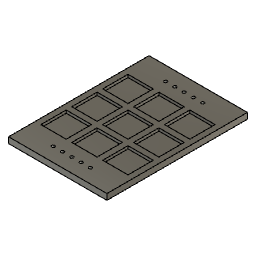
Verkefni_4 (v2~recovered) (Autodesk Fusion 360 design; units mm, degrees)
Autodesk Fusion 360 part; units mm, degrees
sketch "Sketch1" plane through (0, 0, 0) normal (0, 0, 1) x (1, 0, 0)
  line L0 (0, 0) -> (0, 500)
  line L1 (0, 500) -> (350, 500)
  line L2 (350, 500) -> (350, 0)
  line L3 (350, 0) -> (0, 0)
  dimension "d6" = 500
  dimension "d7" = 350
  dimension "d8" = 500
  dimension "d9" = 350
  constraint coincident L0.start L3.end
  constraint vertical L0
  constraint perpendicular L0 L1
  constraint perpendicular L1 L2
  measures "d6" distance of L0.start L0.end
  measures "d7" distance of L0.end L1.end
  measures "d8" distance of L1.end L2.end
  measures "d9" distance of L2.end L0.start
extrude "Extrude1" add sketch "Sketch1" along normal blind 21
sketch "Sketch2" plane through (0, 0, 21) normal (0, 0, 1) x (-1, 0, 0)
  line L0 (-350, 0) -> (-350, -500)
  line L1 (-350, -500) -> (0, -500)
  line L2 (0, -500) -> (0, 0)
  line L3 (0, 0) -> (-350, 0)
  line L4 (0, 0) -> (-20, 0)
  line L5 (-350, 0) -> (-330, 0)
  line L6 (-330, 0) -> (-330, -500)
  line L7 (-20, 0) -> (-20, -500)
  line L8 (-20, -500) -> (-110, -500)
  line L9 (-110, -500) -> (-130, -500)
  line L10 (-130, -500) -> (-220, -500)
  line L11 (-220, -500) -> (-240, -500)
  line L12 (-240, -500) -> (-330, -500)
  line L13 (-110, -500) -> (-110, 0)
  line L14 (-130, -500) -> (-130, 0)
  line L15 (-220, -500) -> (-220, 0)
  line L16 (-240, -500) -> (-240, 0)
  line L17 (0, 0) -> (0, -95)
  line L18 (0, -500) -> (0, -405)
  line L19 (0, -405) -> (-350, -405)
  line L20 (0, -95) -> (-350, -95)
  line L21 (0, -405) -> (0, -315)
  line L22 (0, -315) -> (0, -295)
  line L23 (0, -295) -> (0, -205)
  line L24 (0, -205) -> (0, -185)
  line L25 (0, -185) -> (0, -95)
  line L26 (0, -185) -> (-350, -185)
  line L27 (0, -205) -> (-350, -205)
  line L28 (0, -295) -> (-350, -295)
  line L29 (0, -315) -> (-350, -315)
  dimension "d13" = 20
  dimension "d14" = 500
  dimension "d16" = 90
  dimension "d19" = 20
  dimension "d27" = 95
  dimension "d28" = 95
  dimension "d29" = 350
  dimension "d31" = 90
  dimension "d32" = 20
  dimension "d34" = 90
  dimension "d35" = 20
  constraint coincident L2.end L3.start
  constraint coincident L3 L4.end
  constraint coincident L0.start L3.end
  constraint coincident L3 L5.end
  constraint vertical L6
  constraint vertical L7
  constraint perpendicular L7 L8
  constraint perpendicular L7 L9
  constraint perpendicular L7 L10
  constraint parallel L1 L11
  constraint parallel L1 L12
  constraint perpendicular L9 L13
  constraint perpendicular L8 L14
  constraint perpendicular L1 L15
  constraint perpendicular L11 L16
  constraint parallel L2 L17
  constraint coincident L1.end L2.start
  constraint perpendicular L1 L18
  constraint perpendicular L0 L19
  constraint perpendicular L0 L20
  constraint perpendicular L19 L21
  constraint parallel L2 L22
  constraint coincident L2 L23.end
  constraint coincident L2 L24.end
  constraint coincident L0 L26.end
  constraint perpendicular L0 L26
  constraint coincident L0 L27.end
  constraint perpendicular L0 L27
  constraint coincident L0 L28.end
  constraint perpendicular L0 L28
  constraint coincident L0 L29.end
  constraint perpendicular L0 L29
  measures "d13" distance of L0.start L5.end
  measures "d14" distance of L5.end L6.end
  measures "d16" distance of L7.end L8.end
  measures "d19" distance of L10.end L11.end
  measures "d27" distance of L2.end L17.end
  measures "d28" distance of L1.end L18.end
  measures "d29" distance of L18.end L19.end
  measures "d31" distance of L18.end L21.end
  measures "d32" distance of L21.end L22.end
  measures "d34" distance of L22.end L23.end
  measures "d35" distance of L23.end L24.end
extrude "Extrude2" cut sketch "Sketch2" against normal blind 10 contours L6 L16 L20 L26 | L6 L16 L27 L28 | L14 L15 L20 L26 | L6 L16 L19 L29 | L14 L15 L27 L28 | L7 L13 L20 L26 | L14 L15 L19 L29 | L7 L13 L27 L28 | L7 L13 L19 L29
sketch "Sketch3" plane through (0, 0, 21) normal (0, 0, 1) x (-1, 0, 0)
  line L0 (-330, -95) -> (-240, -95)
  line L1 (-240, -95) -> (-240, -185)
  line L2 (-240, -185) -> (-330, -185)
  line L3 (-330, -185) -> (-330, -95)
  line L4 (-130, -205) -> (-130, -295)
  line L5 (-130, -295) -> (-220, -295)
  line L6 (-220, -295) -> (-220, -205)
  line L7 (-220, -205) -> (-130, -205)
  line L8 (-110, -405) -> (-110, -315)
  line L9 (-110, -315) -> (-20, -315)
  line L10 (-20, -315) -> (-20, -405)
  line L11 (-20, -405) -> (-110, -405)
  line L12 (-110, -295) -> (-110, -205)
  line L13 (-110, -205) -> (-20, -205)
  line L14 (-20, -205) -> (-20, -295)
  line L15 (-20, -295) -> (-110, -295)
  line L16 (-130, -95) -> (-130, -185)
  line L17 (-130, -185) -> (-220, -185)
  line L18 (-220, -185) -> (-220, -95)
  line L19 (-220, -95) -> (-130, -95)
  line L20 (-330, -205) -> (-240, -205)
  line L21 (-240, -205) -> (-240, -295)
  line L22 (-240, -295) -> (-330, -295)
  line L23 (-330, -295) -> (-330, -205)
  line L24 (-130, -315) -> (-130, -405)
  line L25 (-130, -405) -> (-220, -405)
  line L26 (-220, -405) -> (-220, -315)
  line L27 (-220, -315) -> (-130, -315)
  line L28 (-330, -315) -> (-240, -315)
  line L29 (-240, -315) -> (-240, -405)
  line L30 (-240, -405) -> (-330, -405)
  line L31 (-330, -405) -> (-330, -315)
  line L32 (-110, -185) -> (-110, -95)
  line L33 (-110, -95) -> (-20, -95)
  line L34 (-20, -95) -> (-20, -185)
  line L35 (-20, -185) -> (-110, -185)
  line L36 (0, 0) -> (-175, 0)
  circle A0 centre (-175, -50) radius 5.5
  circle A1 centre (-208, -50) radius 5.5
  circle A2 centre (-241, -50) radius 5.5
  circle A3 centre (-142, -50) radius 5.5
  circle A4 centre (-109, -50) radius 5.5
  line L37 (0, -500) -> (-175, -500)
  circle A5 centre (-142, -450) radius 5.5
  circle A6 centre (-109, -450) radius 5.5
  circle A7 centre (-208, -450) radius 5.5
  circle A8 centre (-175, -450) radius 5.5
  circle A9 centre (-241, -450) radius 5.5
  line L38 (-350, 0) -> (-350, -500)
  line L39 (-350, -500) -> (0, -500)
  line L40 (0, -500) -> (0, 0)
  line L41 (0, 0) -> (-350, 0)
  dimension "d43" = 175
  dimension "d44" = 50
  dimension "d46" = 33
  dimension "d55" = 11
  dimension "d56" = 175
  dimension "d57" = 50
  dimension "d60" = 33
  dimension "d64" = 11
  constraint horizontal L36
  constraint coincident L36.start L40.end
  constraint horizontal L37
  measures "d43" distance of L36.start L36.end
  measures "d44" distance of L36.end A0.centre
  measures "d46" distance of A0.centre A1.centre
  measures "d55" diameter of A4
  measures "d56" distance of L37.start L37.end
  measures "d57" distance of L37.end A8.centre
  measures "d60" distance of A7.centre A9.centre
  measures "d64" diameter of A6
extrude "Extrude3" cut sketch "Sketch3" against normal blind 11 contours A0 | A1 | A2 | A3 | A4 | A5 | A6 | A7 | A8 | A9
sketch "Sketch5" plane through (0, 0, 21) normal (0, 0, 1) x (-1, 0, 0)
  circle A0 centre (-175, -50) radius 5.5
  circle A1 centre (-208, -450) radius 5.5
  circle A2 centre (-109, -450) radius 5.5
  circle A3 centre (-241, -450) radius 5.5
  circle A4 centre (-208, -50) radius 5.5
  circle A5 centre (-142, -50) radius 5.5
  circle A6 centre (-175, -450) radius 5.5
  circle A7 centre (-142, -450) radius 5.5
  circle A8 centre (-109, -50) radius 5.5
  circle A9 centre (-241, -50) radius 5.5
  line L0 (-110, -185) -> (-110, -95)
  line L1 (-110, -95) -> (-20, -95)
  line L2 (-20, -95) -> (-20, -185)
  line L3 (-20, -185) -> (-110, -185)
  line L4 (-330, -315) -> (-240, -315)
  line L5 (-240, -315) -> (-240, -405)
  line L6 (-240, -405) -> (-330, -405)
  line L7 (-330, -405) -> (-330, -315)
  line L8 (-130, -315) -> (-130, -405)
  line L9 (-130, -405) -> (-220, -405)
  line L10 (-220, -405) -> (-220, -315)
  line L11 (-220, -315) -> (-130, -315)
  line L12 (-330, -205) -> (-240, -205)
  line L13 (-240, -205) -> (-240, -295)
  line L14 (-240, -295) -> (-330, -295)
  line L15 (-330, -295) -> (-330, -205)
  line L16 (-130, -95) -> (-130, -185)
  line L17 (-130, -185) -> (-220, -185)
  line L18 (-220, -185) -> (-220, -95)
  line L19 (-220, -95) -> (-130, -95)
  line L20 (-110, -295) -> (-110, -205)
  line L21 (-110, -205) -> (-20, -205)
  line L22 (-20, -205) -> (-20, -295)
  line L23 (-20, -295) -> (-110, -295)
  line L24 (-110, -405) -> (-110, -315)
  line L25 (-110, -315) -> (-20, -315)
  line L26 (-20, -315) -> (-20, -405)
  line L27 (-20, -405) -> (-110, -405)
  line L28 (-130, -205) -> (-130, -295)
  line L29 (-130, -295) -> (-220, -295)
  line L30 (-220, -295) -> (-220, -205)
  line L31 (-220, -205) -> (-130, -205)
  line L32 (-330, -95) -> (-240, -95)
  line L33 (-240, -95) -> (-240, -185)
  line L34 (-240, -185) -> (-330, -185)
  line L35 (-330, -185) -> (-330, -95)
  line L36 (-350, 0) -> (-350, -500)
  line L37 (-350, -500) -> (0, -500)
  line L38 (0, -500) -> (0, 0)
  line L39 (0, 0) -> (-350, 0)
equation "lengd = 500 mm" comment "Lengd spilsins"
equation "breydd = 350 mm" comment "Breydd spilsins"
equation "þykkt = 21 mm" comment "Þykkt efnisins"
equation "dypt_holfa = 10 mm" comment "Dýpt hólfanna fyrir leikmenn"
equation "veggir = 20 mm" comment "Stærð skilveggja"
equation "d6 = lengd"
equation "d7 = breydd"
equation "d8 = lengd"
equation "d9 = breydd"
equation "d10 = þykkt"
equation "d13 = veggir"
equation "d14 = lengd"
equation "d16 = ( breydd - veggir ) / 3 - veggir"
equation "d19 = veggir"
equation "d27 = ( ( lengd - breydd ) / 2 ) + veggir"
equation "d28 = ( ( lengd - breydd ) / 2 ) + veggir"
equation "d29 = breydd"
equation "d31 = ( ( breydd - veggir ) / 3 ) - veggir"
equation "d32 = veggir"
equation "d34 = ( ( breydd - veggir ) / 3 ) - veggir"
equation "d35 = veggir"
equation "d36 = -dypt_holfa"
equation "stiga_dýpt = 11 mm" comment "Dýptin á holunum fyrir stiga talninguna"
equation "renna_stiga = 5 mm" comment "Dýptina á rennunum milli staga hólfa"
equation "renna_breydd = 5 mm" comment "Breyddin á rennunni"
equation "d43 = breydd / 2"
equation "d44 = ( lengd / 10 )"
equation "d46 = stiga_dýpt * 3"
equation "d55 = stiga_dýpt"
equation "d56 = breydd / 2"
equation "d57 = lengd / 10"
equation "d60 = stiga_dýpt * 3"
equation "d64 = stiga_dýpt"
equation "d68 = -stiga_dýpt"
